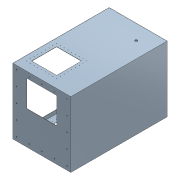
# Autodesk Inventor part: H3NE-B
Saved by Autodesk Inventor 2017 (Build 210142000, 142)
## iProperties
Created: 2016-11-30
Part Number: H3NE-B
Material: Generic
Document SubType Name: Modeling
Designer: krosie
Density: 1 g/cm^3
Appearance: Default
Description: Enclosure Body
Author: krosie
Autodesk Inventor part; units mm, degrees
ref_plane "YZ Plane" through (0, 0, 0) normal (1, 0, 0) x (0, 1, 0)
ref_plane "XZ Plane" through (0, 0, 0) normal (0, 1, 0) x (-1, 0, 0)
ref_plane "XY Plane" through (0, 0, 0) normal (0, 0, 1) x (1, 0, 0)
sketch "Sketch1" plane through (0, 0, 0) normal (0, 1, 0) x (-1, 0, 0)
  line L0 (-381, 431.8) -> (381, 431.8)
  line L1 (381, 431.8) -> (381, -431.8)
  line L2 (381, -431.8) -> (-381, -431.8)
  line L3 (-381, -431.8) -> (-381, 431.8)
  line L4 (-381, 431.8) -> (381, -431.8) construction
  line L5 (381, 431.8) -> (-381, -431.8) construction
  line L6 (384, -434.8) -> (384, 434.8)
  line L7 (384, 434.8) -> (-384, 434.8)
  line L8 (-384, 434.8) -> (-384, -434.8)
  line L9 (-384, -434.8) -> (384, -434.8)
  point P0 (0, 0)
  dimension "d0" = 762
  dimension "d1" = 863.6
  dimension "d2" = 3
  constraints: 20 end point, 4 parallel, 2 midpoint, 2 perpendicular, 1 horizontal, 3 other
  measures "d0" distance of L1.end L2.end
  measures "d1" distance of L0.end L1.end
  measures "d2" distance between parallel lines of L1 L6
extrude "Extrusion1" add sketch "Sketch1" along normal blind 1270
sketch "Sketch2" plane through (0, 1270, 0) normal (0, 1, 0) x (1, 0, 0)
  line L0 (-384, 434.8) -> (-384, -434.8) projected
  line L1 (-384, -434.8) -> (384, -434.8) projected
  line L2 (384, -434.8) -> (384, 434.8) projected
  line L3 (384, 434.8) -> (-384, 434.8) projected
  point P0 (0, 0)
extrude "Extrusion2" add sketch "Sketch2" along normal blind 3
sketch "Sketch3" plane through (0, 0, 0) normal (0, -1, 0) x (1, 0, 0)
  line L0 (-384, 434.8) -> (384, 434.8) projected
  line L1 (-384, -434.8) -> (-384, 434.8) projected
  line L2 (384, -434.8) -> (-384, -434.8) projected
  line L3 (384, 434.8) -> (384, -434.8) projected
  point P0 (0, 0)
extrude "Extrusion3" add sketch "Sketch3" along normal blind 3
sketch "Sketch4" plane through (-384, 1273, -434.8) normal (-1, 0, 0) x (0, 0, 1)
  line L0 (0, 0) -> (869.6, 0) projected
  line L1 (869.6, -1276) -> (869.6, 0) projected
  line L2 (869.6, -1276) -> (0, -1276) projected
  line L3 (0, 0) -> (0, -1276) projected
  line L4 (819.6, -50) -> (50, -50)
  line L5 (50, -50) -> (50, -1226)
  line L6 (50, -1226) -> (819.6, -1226)
  line L7 (819.6, -1226) -> (819.6, -50)
  point P0 (434.8, -1273)
  dimension "d9" = 50
  constraints: 8 end point, 3 other
  measures "d9" distance between parallel lines of L0 L4
extrude "Extrusion4" cut sketch "Sketch4" against normal up to next contours L7 L6 L5 L4
sketch "Sketch5" plane through (-384, 1273, 434.8) normal (0, 0, 1) x (1, 0, 0)
  line L0 (100, -1126) -> (430, -1126)
  line L1 (430, -1126) -> (430, -796)
  line L2 (430, -796) -> (100, -796)
  line L3 (100, -796) -> (100, -1126)
  line L4 (0, -1276) -> (0, 0) projected
  line L5 (768, -1276) -> (0, -1276) projected
  point P0 (384, -1273)
  dimension "d12" = 330
  dimension "d13" = 330
  dimension "d14" = 100
  dimension "d15" = 150
  constraints: 8 end point, 2 parallel, 1 horizontal, 1 perpendicular
  measures "d12" distance of L2.end L1.end
  measures "d13" distance of L1.end L0.end
  measures "d14" distance between parallel lines of L4 L3
  measures "d15" distance between parallel lines of L5 L0
extrude "Extrusion5" cut sketch "Sketch5" against normal through all
sketch "Sketch6" plane through (-384, 1273, 434.8) normal (0, 0, 1) x (1, 0, 0)
  line L0 (100, -796) -> (430, -796) projected
  line L1 (430, -796) -> (430, -1126) projected
  line L2 (430, -1126) -> (100, -1126) projected
  line L3 (100, -1126) -> (100, -796) projected
  line L4 (465, -761) -> (65, -761) construction
  line L5 (65, -761) -> (65, -1161) construction
  line L6 (65, -1161) -> (465, -1161) construction
  line L7 (465, -1161) -> (465, -761) construction
  circle A0 centre (65, -761) radius 2.5
  circle A1 centre (115, -761) radius 2.5
  circle A2 centre (165, -761) radius 2.5
  circle A3 centre (215, -761) radius 2.5
  circle A4 centre (265, -761) radius 2.5
  circle A5 centre (315, -761) radius 2.5
  circle A6 centre (365, -761) radius 2.5
  circle A7 centre (415, -761) radius 2.5
  circle A8 centre (465, -761) radius 2.5
  circle A9 centre (465, -811) radius 2.5
  circle A10 centre (465, -861) radius 2.5
  circle A11 centre (465, -911) radius 2.5
  circle A12 centre (465, -961) radius 2.5
  circle A13 centre (465, -1011) radius 2.5
  circle A14 centre (465, -1061) radius 2.5
  circle A15 centre (465, -1111) radius 2.5
  circle A16 centre (465, -1161) radius 2.5
  circle A17 centre (415, -1161) radius 2.5
  circle A18 centre (365, -1161) radius 2.5
  circle A19 centre (315, -1161) radius 2.5
  circle A20 centre (265, -1161) radius 2.5
  circle A21 centre (215, -1161) radius 2.5
  circle A22 centre (165, -1161) radius 2.5
  circle A23 centre (115, -1161) radius 2.5
  circle A24 centre (65, -1161) radius 2.5
  circle A25 centre (65, -1111) radius 2.5
  circle A26 centre (65, -1061) radius 2.5
  circle A27 centre (65, -1011) radius 2.5
  circle A28 centre (65, -961) radius 2.5
  circle A29 centre (65, -911) radius 2.5
  circle A30 centre (65, -861) radius 2.5
  circle A31 centre (65, -811) radius 2.5
  point P0 (384, -1273)
  point P1 (465, -1158.6)
  point P2 (65, -1158.6)
  dimension "d18" = 35
  dimension "d19" = 5
  dimension "d160" = 50
  dimension "d167" = 50
  dimension "d174" = 50
  dimension "d181" = 50
  constraints: 32 centre point, 8 end point, 2 horizontal, 2 vertical, 1 coincident, 65 other
  measures "d18" distance between parallel lines of L0 L4
  measures "d19" diameter of A0
  measures "d160" distance of A0.centre A1.centre
  measures "d167" distance of A8.centre A9.centre
  measures "d174" distance of A16.centre A17.centre
  measures "d181" distance of A24.centre A25.centre
extrude "Extrusion6" cut sketch "Sketch6" against normal through all contours A0 | A1 | A2 | A3 | A4 | A5 | A6 | A7 | A8 | A9 | A10 | A11 | A12 | A13 | A14 | A15 | A16 | A17 | A18 | A19 | A20 | A21 | A22 | A23 | A24 | A25 | A26 | A27 | A28 | A29 | A30 | A31
fillet "Fillet1" radius 5 4 edges at (-284, 477, -433.3) (-284, 147, -433.3) (46, 147, -433.3) (46, 477, -433.3)
fillet "Fillet2" radius 5 4 edges at (46, 147, 433.3) (46, 477, 433.3) (-284, 147, 433.3) (-284, 477, 433.3)
sketch "Sketch7" plane through (0, -3, 0) normal (0, -1, 0) x (1, 0, 0)
  line L0 (-200, 354.8) -> (200, 354.8)
  line L1 (200, 354.8) -> (200, 4.8)
  line L2 (200, 4.8) -> (-200, 4.8)
  line L3 (-200, 4.8) -> (-200, 354.8)
  line L4 (384, 434.8) -> (-384, 434.8) projected
  line L5 (0, 0) -> (0, 434.8) construction
  dimension "d52" = 400
  dimension "d53" = 350
  dimension "d54" = 80
  constraints: 10 end point, 2 parallel, 1 horizontal, 1 midpoint, 1 perpendicular, 1 other
  measures "d52" distance of L1.end L2.end
  measures "d53" distance of L2.end L0.start
  measures "d54" distance between parallel lines of L4 L0
extrude "Extrusion7" cut sketch "Sketch7" against normal up to surface (3 mm away)
fillet "Fillet3" radius 5 4 edges at (-200, -1.5, 354.8) (200, -1.5, 354.8) (200, -1.5, 4.8) (-200, -1.5, 4.8)
sketch "Sketch8" plane through (0, 1273, 0) normal (0, 1, 0) x (1, 0, 0)
  line L0 (-299, 114) -> (-153, 114)
  line L1 (-151, 112) -> (-151, -112)
  line L2 (-153, -114) -> (-299, -114)
  line L3 (-301, -112) -> (-301, 112)
  line L4 (-301, 114) -> (-151, -114) construction
  line L5 (-151, 114) -> (-301, -114) construction
  line L6 (-381, -431.8) -> (-381, 431.8) projected
  line L7 (0, 0) -> (-381, 0) construction
  arc A0 (-151, 112) -> (-153, 114) centre (-153, 112) ccw
  arc A1 (-153, -114) -> (-151, -112) centre (-153, -112) ccw
  arc A2 (-301, -112) -> (-299, -114) centre (-299, -112) ccw
  arc A3 (-299, 114) -> (-301, 112) centre (-299, 112) ccw
  point P0 (-226, 0)
  dimension "d186" = 150
  dimension "d187" = 228
  dimension "d188" = 80
  dimension "d189" = 2
  constraints: 14 end point, 8 point on circle, 8 point on line, 8 tangent, 4 centre point, 3 equal radius, 3 midpoint, 2 parallel, 1 horizontal, 1 perpendicular, 1 other
  measures "d186" distance of L4.end L5.end
  measures "d187" distance of L5.start L4.end
  measures "d188" distance between parallel lines of L6 L3
  measures "d189" radius of A0
extrude "Extrusion8" cut sketch "Sketch8" against normal up to next
sketch "Sketch10" plane through (0, -3, 0) normal (0, -1, 0) x (1, 0, 0)
  line L0 (-384, 434.8) -> (-384, -434.8) projected
  line L1 (-384, -434.8) -> (384, -434.8) projected
  line L2 (384, 434.8) -> (-384, 434.8) projected
  line L3 (384, -434.8) -> (384, 434.8) projected
  line L4 (334, -384.8) -> (-334, -384.8) construction
  line L5 (-334, -384.8) -> (-334, 384.8) construction
  line L6 (-334, 384.8) -> (334, 384.8) construction
  line L7 (334, 384.8) -> (334, -384.8) construction
  circle A0 centre (-334, -384.8) radius 6
  circle A1 centre (-334, -288.6) radius 6
  circle A2 centre (-334, -192.4) radius 6
  circle A3 centre (-334, -96.2) radius 6
  circle A4 centre (-334, 0) radius 6
  circle A5 centre (-334, 96.2) radius 6
  circle A6 centre (-334, 192.4) radius 6
  circle A7 centre (-334, 288.6) radius 6
  circle A8 centre (-334, 384.8) radius 6
  circle A9 centre (-250.5, -384.8) radius 6
  circle A10 centre (-167, -384.8) radius 6
  circle A11 centre (-83.5, -384.8) radius 6
  circle A12 centre (0, -384.8) radius 6
  circle A13 centre (83.5, -384.8) radius 6
  circle A14 centre (167, -384.8) radius 6
  circle A15 centre (250.5, -384.8) radius 6
  circle A16 centre (334, -384.8) radius 6
  circle A17 centre (-250.5, 384.8) radius 6
  circle A18 centre (-167, 384.8) radius 6
  circle A19 centre (-83.5, 384.8) radius 6
  circle A20 centre (0, 384.8) radius 6
  circle A21 centre (83.5, 384.8) radius 6
  circle A22 centre (167, 384.8) radius 6
  circle A23 centre (250.5, 384.8) radius 6
  circle A24 centre (334, 384.8) radius 6
  circle A25 centre (334, -288.6) radius 6
  circle A26 centre (334, -192.4) radius 6
  circle A27 centre (334, -96.2) radius 6
  circle A28 centre (334, 0) radius 6
  circle A29 centre (334, 96.2) radius 6
  circle A30 centre (334, 192.4) radius 6
  circle A31 centre (334, 288.6) radius 6
  point P0 (0, 0)
  dimension "d91" = 50
  dimension "d92" = 12
  dimension "d95" = 96.2
  dimension "d102" = 83.5
  dimension "d109" = 83.5
  dimension "d116" = 96.2
  constraints: 32 centre point, 8 end point, 2 horizontal, 2 vertical, 1 coincident, 65 other
  measures "d91" distance between parallel lines of L1 L4
  measures "d92" diameter of A0
  measures "d95" distance of A0.centre A1.centre
  measures "d102" distance of A0.centre A9.centre
  measures "d109" distance of A8.centre A17.centre
  measures "d116" distance of A16.centre A25.centre
extrude "Extrusion9" cut sketch "Sketch10" against normal up to surface (3 mm away) contours A0 | A2 | A4 | A6 | A8 | A10 | A12 | A14 | A16 | A18 | A20 | A22 | A24 | A26 | A28 | A30
ref_plane "Work Plane1" through (-384, 1273, 0) normal (0, 0, 1) x (1, 0, 0)
hole "Hole1" at (174, 1073, 434.8) direction (0, 0, -1) diameter 31 end up to face face through (-6.2329, 1018.1606, 431.8) facing (0, 0, -1)
hole "Hole2" at (284, 77, -434.8) direction (0, 0, 1) diameter 12 end up to face face through (-6.2329, 1018.1606, -431.8) facing (0, 0, 1)
equation "\"d48\" = d22"
equation "\"d55\" = d22"
equation "\"d59\" = d22"
equation "\"d121\" = d22"
equation "\"d22\" = 61.35"
body "Solid1"
